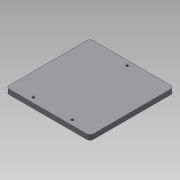
# Autodesk Inventor part: Print Bed
Saved by Autodesk Inventor 2016 (Build 200138000, 138)
## iProperties
Created: 2017-05-15
Part Number: Print Bed
Material: Generic
Document SubType Name: Modeling
Designer: 31745
Density: 1 g/cm^3
Appearance: Default
Author: 31745
Autodesk Inventor part; units mm, degrees
ref_plane "YZ Plane" through (0, 0, 0) normal (1, 0, 0) x (0, 1, 0)
ref_plane "XZ Plane" through (0, 0, 0) normal (0, 1, 0) x (-1, 0, 0)
ref_plane "XY Plane" through (0, 0, 0) normal (0, 0, 1) x (1, 0, 0)
sketch "Sketch1" plane through (0, 0, 0) normal (0, 1, 0) x (-1, 0, 0)
  line L0 (0, 0) -> (-165.1, 0)
  line L1 (-165.1, 0) -> (-165.1, -165.1)
  line L2 (-165.1, -165.1) -> (0, -165.1)
  line L3 (0, -165.1) -> (0, 0)
  dimension "d0" = 165.1
  dimension "d1" = 165.1
  constraints: 8 end point, 2 parallel, 1 horizontal, 1 perpendicular
  measures "d0" distance of L0.start L0.end
  measures "d1" distance of L2.end L0.start
extrude "Extrusion1" add sketch "Sketch1" along normal blind 9.525
fillet "Fillet1" radius 6.35 4 edges at (165.1, 4.7625, 0) (165.1, 4.7625, -165.1) (0, 4.7625, -165.1) (0, 4.7625, 0)
sketch "Sketch4" plane through (0, 9.525, 0) normal (0, 1, 0) x (1, 0, 0)
  arc A0 (0, 6.35) -> (6.35, 0) centre (6.35, 6.35) ccw projected
  line L0 (6.35, 0) -> (158.75, 0) projected
  arc A1 (158.75, 0) -> (165.1, 6.35) centre (158.75, 6.35) ccw projected
  line L1 (165.1, 6.35) -> (165.1, 158.75) projected
  arc A2 (165.1, 158.75) -> (158.75, 165.1) centre (158.75, 158.75) ccw projected
  line L2 (158.75, 165.1) -> (6.35, 165.1) projected
  arc A3 (6.35, 165.1) -> (0, 158.75) centre (6.35, 158.75) ccw projected
  line L3 (0, 158.75) -> (0, 6.35) projected
  line L4 (82.55, 158.75) -> (82.55, 6.35)
  line L5 (82.55, 6.35) -> (6.35, 6.35)
  line L6 (6.35, 6.35) -> (82.55, 6.35)
  line L7 (158.75, 6.35) -> (82.55, 6.35)
  point P0 (0, 0)
  point P1 (82.55, 0)
  dimension "d15" = 6.35
  dimension "d16" = 76.2
  dimension "d18" = 6.35
  constraints: 8 end point, 3 collinear, 1 midpoint, 1 perpendicular, 1 vertical, 1 vertical alignment
  measures "d15" distance between parallel lines of L0 L7
  measures "d16" distance of L7.start L4.end
  measures "d18" distance from line of L2 L4.start
hole "Hole2" at (82.55, 9.525, -158.75) at (158.75, 9.525, -6.35) at (6.35, 9.525, -6.35) direction (0, -1, 0) diameter 4.4958 end through all clearance for "Countersunk Flat Head Screw ISO 2009/7046" size "M4" standard "ISO"
equation "\"d18\" = d15"
body "Solid1"
